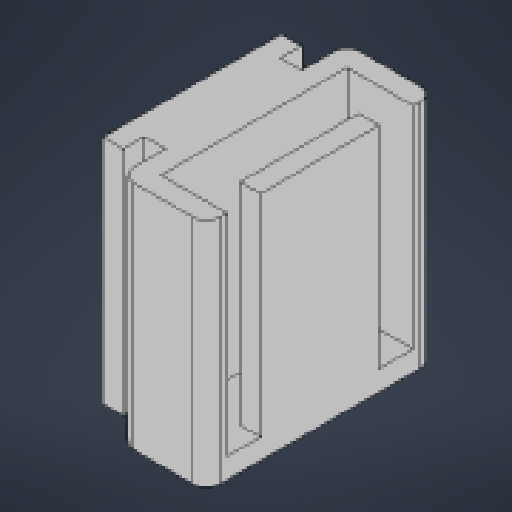
# Autodesk Inventor part: cajaEsp32Cam
Saved by Autodesk Inventor 2026.2 (Build 302298010, 298A)
## iProperties
Created: 2026-08-19
Part Number: cajaEsp32Cam
Material: Genérico
Document SubType Name: Modeling
Designer: samue
Density: 1 g/cm^3
Appearance: Valor por defecto
Author: samue
Autodesk Inventor part; units mm, degrees
ref_plane "YZ Plane" through (0, 0, 0) normal (1, 0, 0) x (0, 1, 0)
ref_plane "XZ Plane" through (0, 0, 0) normal (0, 1, 0) x (-1, 0, 0)
ref_plane "XY Plane" through (0, 0, 0) normal (0, 0, 1) x (1, 0, 0)
sketch "Boceto1" plane through (0, 0, 0) normal (0, 1, 0) x (-1, 0, 0)
  line L0 (0, 0) -> (-6.7, 0)
  line L1 (-6.7, 0) -> (-6.7, -27.4)
  line L2 (-6.7, -27.4) -> (0, -27.4)
  line L3 (0, -27.4) -> (0, 0)
  line L4 (-7.7, 3) -> (1, 3)
  line L5 (3, 1) -> (3, -28.4)
  line L6 (1, -30.4) -> (-7.7, -30.4)
  line L7 (-9.7, -28.4) -> (-9.7, 1)
  arc A0 (3, 1) -> (1, 3) centre (1, 1) ccw
  arc A1 (-7.7, 3) -> (-9.7, 1) centre (-7.7, 1) ccw
  arc A2 (-9.7, -28.4) -> (-7.7, -30.4) centre (-7.7, -28.4) ccw
  arc A3 (1, -30.4) -> (3, -28.4) centre (1, -28.4) ccw
  dimension "d0" = 6.7
  dimension "d1" = 27.4
  dimension "d2" = 3
  dimension "d3" = 2
  constraints: 16 end point, 8 point on circle, 8 tangent, 4 centre point, 4 parallel, 3 equal radius, 2 perpendicular, 1 horizontal, 3 other
  measures "d0" distance of L2.end L1.end
  measures "d1" distance of L1.end L0.end
  measures "d2" distance between parallel lines of L0 L4
  measures "d3" radius of A0
extrude "Extrusión1" add sketch "Boceto1" along normal blind 31
sketch "Boceto2" plane through (0, 0, 0) normal (0, -1, 0) x (1, 0, 0)
  line L0 (9.7, 1) -> (9.7, -28.4) projected
  arc A0 (9.7, 1) -> (7.7, 3) centre (7.7, 1) ccw projected
  line L1 (-1, 3) -> (7.7, 3) projected
  arc A1 (-1, 3) -> (-3, 1) centre (-1, 1) ccw projected
  line L2 (-3, -28.4) -> (-3, 1) projected
  arc A2 (-3, -28.4) -> (-1, -30.4) centre (-1, -28.4) ccw projected
  line L3 (7.7, -30.4) -> (-1, -30.4) projected
  arc A3 (7.7, -30.4) -> (9.7, -28.4) centre (7.7, -28.4) ccw projected
  point P0 (0, 0)
extrude "Extrusión2" add sketch "Boceto2" along normal blind 3
sketch "Boceto3" plane through (9.7, 31, 1) normal (1, 0, 0) x (0, 0, -1)
  line L0 (29.4, -34) -> (29.4, 0) projected
  line L1 (0, 0) -> (29.4, 0) projected
  line L2 (0, -34) -> (0, 0) projected
  line L3 (29.4, -34) -> (0, -34) projected
  line L4 (28.4, -31) -> (28.4, 0) projected
  line L5 (1, -31) -> (1, 0) projected
  line L6 (28.4, -31) -> (1, -31) projected
  line L7 (6, 0) -> (6, -26)
  line L8 (6, -26) -> (23.4, -26)
  line L9 (23.4, -26) -> (23.4, 0)
  line L10 (23.4, -26) -> (23.4, -31)
  line L11 (6, -26) -> (6, -31)
  point P0 (6, 0)
  dimension "d8" = 5
  constraints: 10 end point, 2 perpendicular, 2 point on line, 2 other
  measures "d8" distance between parallel lines of L5 L7
extrude "Extrusión3" cut sketch "Boceto3" against normal blind 3 contours L4 L6 L10 L9 L1 | L1 L7 L11 L6 L5
sketch "Boceto4" plane through (0, -3, 0) normal (0, -1, 0) x (1, 0, 0)
  line L0 (-3, 1) -> (-3, -28.4) projected
  line L1 (-3, -3.7) -> (-6.1, -3.7)
  line L2 (-6.1, -3.7) -> (-6.1, -0.6)
  line L3 (-6.1, -0.6) -> (-9.1, -0.6)
  line L4 (-3, -23.7) -> (-6.1, -23.7)
  line L5 (-6.1, -23.7) -> (-6.1, -26.8)
  line L6 (-6.1, -26.8) -> (-9.1, -26.8)
  line L7 (-9.1, -26.8) -> (-9.1, -0.6)
  line L8 (0, 0) -> (0, -27.4) projected
  point P0 (0, -13.7)
  dimension "d11" = 3.1
  dimension "d12" = 3.1
  dimension "d13" = 3
  dimension "d14" = 3.1
  dimension "d15" = 10
  dimension "d16" = 10
  dimension "d17" = 3.1
  constraints: 14 end point, 7 perpendicular, 2 point on line, 1 midpoint
  measures "d11" distance of L1.start L1.end
  measures "d12" distance of L1.end L2.end
  measures "d13" distance of L2.end L3.end
  measures "d14" distance of L4.end L5.end
  measures "d15" distance from line of point (0, -13.7) L1
  measures "d16" distance from line of point (0, -13.7) L4
  measures "d17" distance between parallel lines of L0 L5
extrude "Extrusión4" add sketch "Boceto4" against normal up to surface (34 mm away)
sketch "Boceto5" plane through (0, -3, 0) normal (0, -1, 0) x (1, 0, 0)
  line L0 (9.7, 0) -> (0, 0) projected
  line L1 (9.7, -5) -> (9.7, 0) projected
  line L2 (9.7, -5) -> (6.7, -5) projected
  line L3 (6.7, -22.4) -> (6.7, -5) projected
  line L4 (9.7, -22.4) -> (6.7, -22.4) projected
  line L5 (9.7, -27.4) -> (9.7, -22.4) projected
  line L6 (0, -27.4) -> (9.7, -27.4) projected
  line L7 (0, 0) -> (0, -27.4) projected
  point P0 (2.5, -2.5)
  point P1 (2.5, -24.9)
  dimension "d20" = 2.5
  dimension "d21" = 2.5
  measures "d20" distance from line of L0 point (2.5, -2.5)
  measures "d21" distance from line of L7 point (2.5, -2.5)
hole "Agujero1" at (2.5, -3, -2.5) at (2.5, -3, -24.9) direction (0, 1, 0) diameter 4.5 end through all
